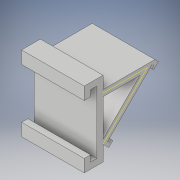
# Autodesk Inventor part: Substrategrip45degreesThick
Saved by Autodesk Inventor 2019 (Build 230136000, 136)
## iProperties
Created: 2018-09-07
Part Number: Substrategrip45degreesThick
Material: Generic
Document SubType Name: Modeling
Designer: s152529
Density: 1 g/cm^3
Appearance: Default
Author: s152529
Autodesk Inventor part; units mm, degrees
ref_plane "XZ Plane" through (0, 0, 0) normal (0, 1, 0) x (-1, 0, 0)
ref_plane "XY Plane" through (0, 0, 0) normal (0, 0, 1) x (1, 0, 0)
sketch "Sketch1" plane through (0, 0, 0) normal (0, 0, 1) x (1, 0, 0)
  line L0 (-25, 30) -> (25, 30)
  line L1 (25, 30) -> (25, -30)
  line L2 (25, -30) -> (-25, -30)
  line L3 (-25, -30) -> (-25, 30)
  point P0 (0, 0)
  dimension "d0" = 50
  dimension "d1" = 60
  dimension "d2" = 30
  dimension "d3" = 25
  constraints: 8 end point, 2 parallel, 1 horizontal, 1 perpendicular
  measures "d0" distance of L1.end L2.end
  measures "d1" distance between parallel lines of L2 L0
  measures "d2" distance from line of L0 point (0, 0)
  measures "d3" distance from line of point (0, 0) L3
extrude "Extrusion1" add sketch "Sketch1" along normal blind 5
sketch "Sketch2" plane through (0, 0, 5) normal (0, 0, 1) x (1, 0, 0)
  line L0 (-25, 30) -> (-25, -30) projected
  line L1 (-25, 25) -> (25, 25)
  line L2 (25, -30) -> (25, 30) projected
  line L3 (25, 30) -> (-25, 30) projected
  point P0 (0, 0)
  dimension "d6" = 5
  constraints: 2 end point, 2 point on line, 1 horizontal
  measures "d6" distance between parallel lines of L3 L1
extrude "Extrusion2" add sketch "Sketch2" along normal blind 10
sketch "Sketch3" plane through (0, 0, 5) normal (0, 0, 1) x (1, 0, 0)
  line L0 (-25, -30) -> (-25, 30) projected
  line L1 (-25, -25) -> (25, -25)
  line L2 (25, 30) -> (25, -30) projected
  line L3 (-25, -30) -> (25, -30) projected
  point P0 (0, 0)
  dimension "d9" = 5
  constraints: 2 end point, 2 point on line, 1 horizontal
  measures "d9" distance between parallel lines of L3 L1
extrude "Extrusion3" add sketch "Sketch3" along normal blind 10
sketch "Sketch4" plane through (-25, -25, 5) normal (0, 1, 0) x (1, 0, 0)
  line L0 (0, 5) -> (0, -10) projected
  line L1 (0, -5) -> (50, -5)
  line L2 (50, 5) -> (50, -10) projected
  line L3 (0, -10) -> (50, -10) projected
  point P0 (25, 5)
  dimension "d12" = 5
  constraints: 2 end point, 2 point on line, 1 horizontal
  measures "d12" distance between parallel lines of L3 L1
extrude "Extrusion4" add sketch "Sketch4" along normal blind 5
sketch "Sketch5" plane through (-25, 25, 5) normal (0, -1, 0) x (1, 0, 0)
  line L0 (0, -5) -> (0, 10) projected
  line L1 (0, 5) -> (50, 5)
  line L2 (50, -5) -> (50, 10) projected
  line L3 (50, 10) -> (0, 10) projected
  point P0 (25, -5)
  dimension "d15" = 5
  constraints: 2 end point, 2 point on line, 1 horizontal
  measures "d15" distance between parallel lines of L3 L1
extrude "Extrusion5" add sketch "Sketch5" along normal blind 5
ref_plane "Work Plane1" through (25, 30, 15) normal (1, 0, 0) x (0, 1, 0)
sketch "Sketch6" plane through (25, 30, 15) normal (1, 0, 0) x (0, 1, 0)
  line L0 (0, -15) -> (-60, -15) projected
  line L1 (-47.6803, -15) -> (-12.325, -50.3553)
  line L2 (-47.6803, -15) -> (2.3197, -15) construction
  line L3 (-12.325, -50.3553) -> (-12.325, -15)
  line L4 (0, -15) -> (0, 0) projected
  point P0 (-30, -15)
  dimension "d18" = 50
  dimension "d19" = 45
  dimension "d36" = 12.325
  constraints: 6 end point, 2 point on line, 1 equal length, 1 horizontal, 1 perpendicular
  measures "d18" distance of L1.start L1.end
  measures "d19" angle of L1 L2
  measures "d36" distance between parallel lines of L4 L3
surface extrude "ExtrusionSrf1" sketch "Sketch6" against normal up to surface (50 mm away) shown yes curves L1 L3
sketch "Sketch7" plane through (-25, -17.6803, 0) normal (0, 0.7071068, 0.7071068) x (1, 0, 0)
  point P0 (25, 12.5019)
thicken "Thicken1" operation add thickness 5 both sides yes extend neighbours no toward (0, 1, 0) faces at (8.3333, 17.675, -23.5702) (8.3333, -5.8952, -11.7851)
sketch "Sketch8" plane through (25, 20.175, -41.3909) normal (0, -0.7071068, -0.7071068) x (-1, 0, 0)
  line L0 (0, 0) -> (0, -29.2678) projected
  line L1 (0, -3.3808) -> (0, -53.3808)
  line L2 (0, -53.3808) -> (50, -53.3808)
  line L3 (50, -29.3915) -> (50, -64.7468) projected
  line L4 (0, -3.3808) -> (50, -3.3808)
  line L5 (50, -29.2678) -> (50, 0) projected
  line L6 (0, 0) -> (50, 0)
  line L7 (50, 0) -> (50, -3.3808)
  line L8 (50, -3.3808) -> (0, -3.3808)
  line L9 (0, -3.3808) -> (0, 0)
  point P0 (25, -43.5336)
  dimension "d37" = 50
  constraints: 14 end point, 3 point on line, 2 horizontal, 2 parallel, 2 perpendicular, 1 collinear
  measures "d37" distance of L1.start L1.end
extrude "Extrusion10" add sketch "Sketch8" along normal blind 4
sketch "Sketch13" plane through (25, -19.4481, -1.7678) normal (0, -0.7071068, -0.7071068) x (-1, 0, 0)
  line L0 (0, -8.7113) -> (0, 26.644) projected
  line L1 (50, 0) -> (0, 0) projected
  line L2 (0, 2.6469) -> (50, 2.6469)
  line L3 (50, 2.6469) -> (50, 0)
  line L4 (50, 0) -> (0, 0)
  line L5 (0, 0) -> (0, 2.6469)
  point P0 (25, 12.5019)
  constraints: 8 end point, 2 parallel, 1 horizontal, 1 perpendicular, 1 point on line
extrude "Extrusion11" add sketch "Sketch13" along normal blind 4
sketch "Sketch15" plane through (-25, 17.7844, -39.0003) normal (0, -0.7071068, 0.7071068) x (1, 0, 0)
  line L0 (50, 0) -> (50, -4) projected
  line L1 (50, -2) -> (0, -2)
  line L2 (0, 0) -> (0, -4) projected
  line L3 (50, -4) -> (0, -4)
  line L4 (0, -4) -> (0, -2)
  line L5 (0, -2) -> (50, -2)
  line L6 (50, -2) -> (50, -4)
  point P0 (25, 15.0019)
  constraints: 10 end point, 2 midpoint, 2 parallel, 1 horizontal, 1 perpendicular
extrude "Extrusion12" add sketch "Sketch15" along normal blind 2
sketch "Sketch19" plane through (25, -17.5764, -3.6394) normal (0, 0.7071068, -0.7071068) x (-1, 0, 0)
  line L0 (0, -4) -> (50, -4) projected
  line L1 (50, -6.2113) -> (50, 2.5) projected
  line L2 (0, -4) -> (50, -4)
  line L3 (50, -4) -> (50, -2)
  line L4 (50, -2) -> (0, -2)
  line L5 (0, -2) -> (0, -4)
  point P0 (25, 15.0019)
  dimension "d44" = 2
  constraints: 8 end point, 2 parallel, 1 horizontal, 1 perpendicular, 1 point on line
  measures "d44" distance of L3.end L2.end
extrude "Extrusion13" add sketch "Sketch19" along normal blind 2
body "Solid1"
body "Srf1"
